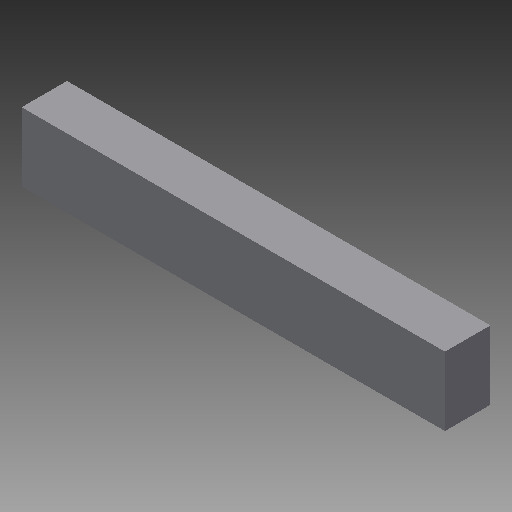
# Autodesk Inventor part: snapPinout
Saved by Autodesk Inventor 2017 (Build 210142000, 142)
## iProperties
Created: 2016-08-31
Part Number: snapPinout
Material: Generic
Document SubType Name: Modeling
Designer: Zara
Density: 1 g/cm^3
Appearance: Default
Author: Zara
Autodesk Inventor part; units mm, degrees
ref_plane "YZ Plane" through (0, 0, 0) normal (1, 0, 0) x (0, 1, 0)
ref_plane "XZ Plane" through (0, 0, 0) normal (0, 1, 0) x (-1, 0, 0)
ref_plane "XY Plane" through (0, 0, 0) normal (0, 0, 1) x (1, 0, 0)
sketch "Sketch1" plane through (0, 0, 0) normal (0, 1, 0) x (-1, 0, 0)
  line L0 (-25.654, 2.7559) -> (25.654, 2.7559)
  line L1 (25.654, 2.7559) -> (25.654, -2.7559)
  line L2 (25.654, -2.7559) -> (-25.654, -2.7559)
  line L3 (-25.654, -2.7559) -> (-25.654, 2.7559)
  line L4 (-25.654, 2.7559) -> (25.654, -2.7559) construction
  line L5 (25.654, 2.7559) -> (-25.654, -2.7559) construction
  point P0 (0, 0)
  dimension "d0" = 51.308
  dimension "d1" = 5.5118
  constraints: 12 end point, 2 midpoint, 2 parallel, 1 horizontal, 1 perpendicular
  measures "d0" distance of L1.end L2.end
  measures "d1" distance of L2.end L0.start
extrude "Extrusion1" add sketch "Sketch1" along normal blind 8.3312
body "Solid1"
